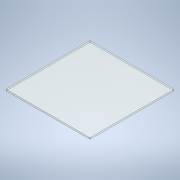
# Autodesk Inventor part: GlassBed
Saved by Autodesk Inventor 2020.2 (Build 242310000, 310)
## iProperties
Created: 2020-07-29
Part Number: GlassBed
Material: Glass
Document SubType Name: Modeling
Designer: JK
Density: 2.18 g/cm^3
Appearance: Clear
Author: JK
Autodesk Inventor part; units mm, degrees
ref_plane "YZ Plane" through (0, 0, 0) normal (1, 0, 0) x (0, 1, 0)
ref_plane "XZ Plane" through (0, 0, 0) normal (0, 1, 0) x (-1, 0, 0)
ref_plane "XY Plane" through (0, 0, 0) normal (0, 0, 1) x (1, 0, 0)
sketch "Sketch1" plane through (0, 0, 0) normal (0, 1, 0) x (-1, 0, 0)
  line L0 (-117.5, 117.5) -> (117.5, 117.5)
  line L1 (117.5, 117.5) -> (117.5, -117.5)
  line L2 (117.5, -117.5) -> (-117.5, -117.5)
  line L3 (-117.5, -117.5) -> (-117.5, 117.5)
  line L4 (-117.5, 117.5) -> (117.5, -117.5) construction
  line L5 (117.5, 117.5) -> (-117.5, -117.5) construction
  point P0 (0, 0)
  dimension "d0" = 235
  dimension "d1" = 235
  constraints: 12 end point, 2 midpoint, 2 parallel, 1 horizontal, 1 perpendicular
  measures "d0" distance of L0.end L1.end
  measures "d1" distance of L1.end L2.end
extrude "Extrusion1" add sketch "Sketch1" along normal blind 4
fillet "Fillet1" radius 2 4 edges at (117.5, 2, 117.5) (117.5, 2, -117.5) (-117.5, 2, -117.5) (-117.5, 2, 117.5)
body "Solid1"
